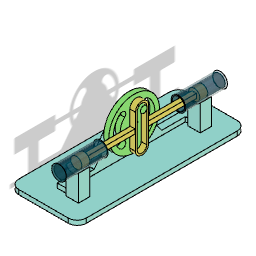
Scotch-Yoke_Mechanism (Autodesk Fusion 360 design; units mm, degrees)
Autodesk Fusion 360 part; units mm, degrees
note: some values were not read from the file. Set by a fixed rule: which sketch regions a step uses.
sketch "stand" plane through (0, 0, 0) normal (0, 0, 1) x (1, 0, 0) in component "holder stand"
  line L0 (75, 30) -> (-75, 30)
  line L1 (-75, 30) -> (-75, -30)
  line L2 (-75, -30) -> (75, -30)
  line L3 (75, -30) -> (75, 30)
  line L4 (75, 30) -> (-75, -30) construction
  line L5 (-75, 30) -> (75, -30) construction
  circle A0 centre (-61.0686, -17.8895) radius 7.5
  line L6 (0, 0) -> (75, 0)
  circle A1 centre (-61.0686, 17.8895) radius 7.5
  circle A2 centre (61.0686, 17.8895) radius 7.5
  circle A3 centre (61.0686, -17.8895) radius 7.5
  line L7 (20, 0) -> (-20, 0)
  line L8 (-20, 6) -> (20, 6)
  line L9 (-20, 0) -> (-30, 0)
  line L10 (-30, 0) -> (-30, 6)
  line L11 (-30, 6) -> (-20, 6)
  line L12 (20, 0) -> (30, 0)
  line L13 (30, 0) -> (30, 6)
  line L14 (30, 6) -> (20, 6)
  dimension "d1" = 150
  dimension "d2" = 60
  dimension "d3" = 15
  dimension "d10" = 40
  dimension "d11" = 6
  dimension "d16" = 40
  constraint horizontal L0
  constraint perpendicular L0 L1
  constraint parallel L0 L2
  constraint parallel L1 L3
  constraint coincident L4 L6.start
  constraint coincident L5 L6.start
  constraint midpoint L3 L6.end
  constraint symmetric A0 L6 A1
  constraint horizontal L7
  constraint horizontal L8
  constraint coincident L6 L7.start
  constraint horizontal L9
  constraint vertical L10
  constraint horizontal L11
  constraint horizontal L12
  constraint vertical L13
  constraint horizontal L14
  measures "d1" distance of L1.end L2.end
  measures "d2" distance of L0.end L1.end
  measures "d3" diameter of A0
  measures "d10" distance of L7.start L7.end
  measures "d11" distance of L7.start L8.end
  measures "d16" distance of L7.start L7.end
extrude "Extrude1" add sketch "stand" along normal blind 4 contours A0 | A1 | A2 | A3 makes body 1 at (68.5593, -18.2634, 2.6667) makes body 2 at (-53.5779, -18.2634, 2.6667) makes body 3 at (68.5593, 17.5157, 2.6667) makes body 4 at (-53.5779, 17.5157, 2.6667) in component "holder stand"
extrude "Extrude2" add sketch "stand" along normal blind 8 and the other way blind -4 contours L0 L1 L2 L3 | A0 | L6 L7 L8 L9 L10 L11 L12 L13 L14 | A1 | A2 | A3 bodies 1 2 3 4 in component "holder stand"
extrude "Extrude3" cut sketch "stand" along normal blind 50 contours L6 L7 L8 L9 L10 L11 L12 L13 L14 bodies 1 in component "holder stand"
fillet "Fillet1" radius 8 4 edges at (75, -30, 6) (-75, -30, 6) (75, 30, 6) (-75, 30, 6) on bodies 1 in component "holder stand"
sketch "holder" plane through (0, -6.0574, 0) normal (0, 1, 0) x (-1, 0, 0) in component "holder"
  line L0 (-30, 4) -> (30, 4)
  line L1 (30, 4) -> (30, 8)
  line L2 (30, 8) -> (-30, 8)
  line L3 (-30, 8) -> (-30, 4)
  line L4 (-30, 4) -> (30, 4)
  line L5 (30, 4) -> (30, 12)
  line L6 (30, 12) -> (-30, 12)
  line L7 (-30, 12) -> (-30, 4)
  line L8 (-30, 12) -> (-4.0576, 46.088)
  line L9 (30, 12) -> (4.0576, 46.088)
  arc A0 (4.0576, 46.088) -> (-4.0576, 46.088) centre (0, 43) ccw
  circle A1 centre (0, 35) radius 3
  line L10 (30, 12) -> (30, 8)
  line L11 (-30, 12) -> (-30, 4)
  dimension "d19" = 6
  constraint horizontal L4
  constraint vertical L5
  constraint horizontal L6
  constraint vertical L7
  constraint coincident L0.start L3.end
  constraint tangent L8 A0
  constraint coincident L1.end L2.start
  measures "d19" diameter of A1
extrude "Extrude1'" add sketch "holder" along normal blind 6 separate body contours L0 L1 L2 L3 L4 L5 L7 L11 | L2 L5 L6 L7 L10 L11 | L6 L8 L9 A0 | A1 makes body 5 in component "holder"
extrude "Extrude2'" add sketch "holder" along normal blind 12 contours A1 bodies 5 in component "holder"
sketch "crank" plane through (0, 5.9426, 0) normal (0, 1, 0) x (-1, 0, 0) in component "crank"
  circle A0 centre (0, 35) radius 3
  circle A1 centre (0, 35) radius 22.5
  circle A2 centre (0, 50) radius 3
  arc A3 (-8.4317, 44.0502) -> (-12.5322, 48.4516) centre (-10.4819, 46.2509) ccw
  arc A4 (-12.5322, 21.5484) -> (-8.4317, 25.9498) centre (-10.4819, 23.7491) ccw
  arc A5 (-8.4317, 44.0502) -> (-8.4317, 25.9498) centre (0, 35) ccw
  arc A6 (12.5322, 21.5484) -> (12.5322, 48.4516) centre (0, 35) ccw
  arc A7 (-12.5322, 48.4516) -> (-12.5322, 21.5484) centre (0, 35) ccw
  arc A8 (8.4317, 25.9498) -> (8.4317, 44.0502) centre (0, 35) ccw
  arc A9 (12.5322, 48.4516) -> (8.4317, 44.0502) centre (10.4819, 46.2509) ccw
  arc A10 (8.4317, 25.9498) -> (12.5322, 21.5484) centre (10.4819, 23.7491) ccw
  dimension "d22" = 45
  dimension "d23" = 6
  constraint concentric A0 A1
  constraint concentric A0 A5
  constraint concentric A1 A6
  constraint tangent A5 A9
  constraint coincident A3.end A6
  constraint concentric A5 A8
  constraint concentric A6 A7
  measures "d22" diameter of A1
  measures "d23" diameter of A2
extrude "Extrude1''" add sketch "crank" along normal blind -5 and the other way blind 0.5 separate body makes body 6 in component "crank"
extrude "Extrude2''" add sketch "crank" along normal blind 7 and the other way blind 5 contours A2 bodies 6 in component "crank"
sketch "slider" plane through (0, 5.4426, 0) normal (0, 1, 0) x (-1, 0, 0) in component "slider"
  arc A0 (-8.4317, 44.0502) -> (-12.5322, 48.4516) centre (-10.4819, 46.2509) ccw
  arc A1 (-8.4317, 44.0502) -> (-8.4317, 25.9498) centre (0, 35) ccw
  arc A2 (-12.5322, 21.5484) -> (-8.4317, 25.9498) centre (-10.4819, 23.7491) ccw
  arc A3 (-12.5322, 48.4516) -> (-12.5322, 21.5484) centre (0, 35) ccw
  arc A4 (8.4317, 25.9498) -> (12.5322, 21.5484) centre (10.4819, 23.7491) ccw
  arc A5 (8.4317, 25.9498) -> (8.4317, 44.0502) centre (0, 35) ccw
  arc A6 (12.5322, 48.4516) -> (8.4317, 44.0502) centre (10.4819, 46.2509) ccw
  arc A7 (12.5322, 21.5484) -> (12.5322, 48.4516) centre (0, 35) ccw
  circle A8 centre (0, 50) radius 3
  circle A9 centre (0, 35) radius 3
  circle A10 centre (0, 35) radius 22.5
  line L0 (-5.8308, 50.0372) -> (-5.831, 20)
  line L1 (5.831, 20) -> (5.831, 50)
  line L2 (4.2426, 20) -> (4.2426, 50)
  line L3 (-4.2426, 20) -> (-4.2426, 50)
  arc A11 (5.831, 50) -> (-5.8308, 49.9628) centre (0, 50) ccw
  arc A12 (4.2426, 50) -> (-4.2426, 50) centre (0, 50) ccw
  arc A13 (-5.831, 20) -> (5.831, 20) centre (0, 20) ccw
  arc A14 (-4.2426, 20) -> (4.2426, 20) centre (0, 20) ccw
  constraint concentric A8 A12
  constraint concentric A11 A12
  constraint coincident L0.start A11
  constraint tangent L0 A13
  constraint tangent L1 A11
  constraint vertical L1
  constraint tangent L2 A12
  constraint parallel L1 L2
  constraint tangent L3 A12
  constraint parallel L2 L3
  constraint coincident L0 A11.end
extrude "Extrude1'''" add sketch "slider" along normal blind 7 and the other way blind -2 separate body contours L0 L1 A11 A13 makes body 7 in component "slider"
sketch "slider right" plane through (-5.831, 0, 0) normal (-1, 0, 0) x (0, -1, 0) in component "slider"
  line L0 (-7.4426, 20) -> (-7.4426, 50)
  line L1 (-7.4426, 50) -> (-12.4426, 50)
  line L2 (-12.4426, 50) -> (-12.4426, 20)
  line L3 (-12.4426, 20) -> (-7.4426, 20)
  line L4 (-7.9426, 33) -> (-11.9426, 33)
  line L5 (-11.9426, 33) -> (-11.9426, 37)
  line L6 (-11.9426, 37) -> (-7.9426, 37)
  line L7 (-7.9426, 37) -> (-7.9426, 33)
  line L8 (-7.9426, 33) -> (-11.9426, 37) construction
  line L9 (-11.9426, 33) -> (-7.9426, 37) construction
  circle A0 centre (-9.9426, 35) radius 3
  dimension "d36" = 4
  dimension "d76" = 6
  constraint horizontal L4
  constraint perpendicular L4 L5
  constraint parallel L4 L6
  constraint parallel L5 L7
  constraint midpoint L9 A0.centre
  measures "d36" distance of L5.end L6.end
  measures "d76" diameter of A0
sketch "slider left" plane through (5.831, 0, 0) normal (1, 0, 0.000004) x (0, 1, 0) in component "slider"
  line L0 (7.4426, 50.0372) -> (7.4426, 20)
  line L1 (7.4426, 20) -> (12.4426, 20)
  line L2 (12.4426, 20) -> (12.4426, 50.0372)
  line L3 (12.4426, 50.0372) -> (7.4426, 50.0372)
  line L4 (11.9426, 33.0186) -> (7.9426, 33.0186)
  line L5 (7.9426, 33.0186) -> (7.9426, 37.0186)
  line L6 (7.9426, 37.0186) -> (11.9426, 37.0186)
  line L7 (11.9426, 37.0186) -> (11.9426, 33.0186)
  line L8 (11.9426, 33.0186) -> (7.9426, 37.0186) construction
  line L9 (7.9426, 33.0186) -> (11.9426, 37.0186) construction
  dimension "d37" = 4
  dimension "d38" = 4
  constraint horizontal L4
  constraint perpendicular L4 L5
  constraint parallel L4 L6
  constraint parallel L5 L7
  measures "d37" distance of L5.end L6.end
  measures "d38" distance of L4.end L5.end
extrude "Extrude2'''" add sketch "slider right" along normal blind 50 contours L4 L5 L6 L7 bodies 7 in component "slider"
extrude "Extrude3'" add sketch "slider left" along normal blind 50 contours L4 L5 L6 L7 bodies 7 in component "slider"
extrude "Extrude3''" add 1 faces at (0.5, 12.9426, 48.2662) along direction (0, 1, 0) blind 1 on bodies 6 bodies 6 in component "crank"
move_face "OffsetFaces1" offset -0.3 1 faces at (-2.9851, 1.9426, 35.2987) on bodies 5 in component "holder"
sketch "piston" plane through (5.831, 0, 0) normal (1, 0, 0.000004) x (0, 1, 0) in component "slider"
  line L0 (11.9426, 37.0186) -> (11.9426, 33.0186)
  line L1 (11.9426, 33.0186) -> (7.9426, 33.0186)
  line L2 (7.9426, 33.0186) -> (7.9426, 37.0186)
  line L3 (7.9426, 37.0186) -> (11.9426, 37.0186)
  line L4 (7.4426, 50.0372) -> (7.4426, 20)
  line L5 (7.4426, 20) -> (12.4426, 20)
  line L6 (12.4426, 20) -> (12.4426, 50.0372)
  line L7 (12.4426, 50.0372) -> (7.4426, 50.0372)
  circle A0 centre (9.9426, 35.0186) radius 3
  dimension "d71" = 6
  measures "d71" diameter of A0
extrude "Extrude4" add sketch "piston" along normal blind 50 and the other way blind -43 contours L0 L1 L2 L3 | L4 L6 A0 | L4 A0 | L6 A0 bodies 7 in component "slider"
extrude "Extrude5" add sketch "slider right" along normal blind 50 and the other way blind -43 contours L0 L2 A0 | L0 A0 | L2 A0 | L4 L5 L6 L7 bodies 7 in component "slider"
move_face "OffsetFaces1'" offset 2 1 faces at (53.4976, 12.9277, 35.3175) on bodies 7 in component "slider"
move_face "OffsetFaces2" offset 2 1 faces at (-51.1643, 6.9464, 35.1495) on bodies 7 in component "slider"
sketch "Sketch1" plane through (-55.7663, 0, 0) normal (-1, 0, 0) x (0, -1, 0) in component "right cylinder"
  circle A0 centre (-9.9426, 35) radius 5
  circle A1 centre (-9.9426, 35) radius 5.5
  circle A2 centre (-9.9426, 35) radius 6.5
  dimension "d84" = 11
  dimension "d85" = 13
  constraint concentric A0 A1
  constraint concentric A1 A2
  measures "d84" diameter of A1
  measures "d85" diameter of A2
extrude "Extrude1''''" add sketch "Sketch1" along normal blind 16 and the other way blind -15 separate body contours A0 makes body 8 in component "right cylinder"
extrude "Extrude2''''" add sketch "Sketch1" along normal blind 16 and the other way blind 21 separate body contours A2 makes body 9 in component "right cylinder"
extrude "Extrude3'''" add sketch "Sketch1" along normal blind 16 and the other way blind -15 contours A1 bodies 8 9 in component "right cylinder"
sketch "Sketch1 (2)" plane through (69.5884, 0, 0.0003) normal (1, 0, 0.000004) x (0, 1, 0) in component "left cylinder"
  circle A0 centre (9.9426, 35.0185) radius 5
extrude "Extrude1'''''" add 1 faces at (-34.7663, 3.8002, 34.6771) along direction (1, 0, 0) blind 106 and the other way blind -69 separate body on bodies 8 makes body 10 in component "left cylinder"
sketch "Sketch2" plane through (71.2337, 0, 0) normal (1, 0, 0) x (0, 1, 0) in component "left cylinder"
  circle A0 centre (9.9426, 35) radius 5.5
  circle A1 centre (9.9426, 35) radius 6.5
  circle A2 centre (9.9426, 35) radius 6.5
  constraint concentric A0 A2
extrude "Extrude2'''''" add sketch "Sketch2" against normal blind 1 contours A0 | A1 A2 bodies 10 in component "left cylinder"
sketch "Sketch5" plane through (0, 0, 8) normal (0, 0, 1) x (-1, 0, 0) in component "holder"
  arc A0 (-67, 30.0574) -> (-75, 22.0574) centre (-67, 22.0574) ccw
  line L0 (-75, 22.0574) -> (-75, -21.9426)
  arc A1 (-75, -21.9426) -> (-67, -29.9426) centre (-67, -21.9426) ccw
  line L1 (-67, -29.9426) -> (67, -29.9426)
  arc A2 (67, -29.9426) -> (75, -21.9426) centre (67, -21.9426) ccw
  line L2 (75, -21.9426) -> (75, 22.0574)
  arc A3 (75, 22.0574) -> (67, 30.0574) centre (67, 22.0574) ccw
  line L3 (67, 30.0574) -> (-67, 30.0574)
  line L4 (-30, 0.0574) -> (-30, 6.0574)
  line L5 (-30, 6.0574) -> (30, 6.0574)
  line L6 (30, 6.0574) -> (30, 0.0574)
  line L7 (30, 0.0574) -> (-30, 0.0574)
  line L8 (30, 0.0574) -> (50.8975, 0.0574)
  line L9 (56.8975, 0.0574) -> (56.8975, 6.0574)
  line L10 (56.8975, 6.0574) -> (30, 6.0574)
  line L11 (30, 6.0574) -> (30, 0.0574)
  line L12 (50.8975, 0.0574) -> (50.8975, -12.9426)
  line L13 (50.8975, -12.9426) -> (56.8975, -12.9426)
  line L14 (56.8975, -12.9426) -> (56.8975, 0.0574)
  line L15 (0, 6.0574) -> (0, 0)
  line L16 (-56.8975, 6.0574) -> (-30, 6.0574)
  line L17 (-30, 0.0574) -> (-50.8975, 0.0574)
  line L18 (-56.8975, 0.0574) -> (-56.8975, 6.0574)
  line L19 (-50.8975, 0.0574) -> (-50.8975, -12.9426)
  line L20 (-56.8975, -12.9426) -> (-56.8975, 0.0574)
  line L21 (-50.8975, -12.9426) -> (-56.8975, -12.9426)
  line L22 (-59, -15) -> (-49, -15)
  line L23 (-49, -15) -> (-49, -4)
  line L24 (-49, -4) -> (-59, -4)
  line L25 (-59, -4) -> (-59, -15)
  line L26 (0, -25) -> (0, -5)
  line L27 (49, -4) -> (59, -4)
  line L28 (49, -15) -> (49, -4)
  line L29 (59, -15) -> (49, -15)
  line L30 (59, -4) -> (59, -15)
  dimension "d107" = 6
  dimension "d108" = 13
  constraint horizontal L8
  constraint vertical L9
  constraint horizontal L10
  constraint vertical L11
  constraint coincident L6.end L7.start
  constraint vertical L12
  constraint horizontal L13
  constraint vertical L14
  constraint midpoint L5 L15.start
  constraint coincident L15.end origin
  constraint symmetric L6.end L15 L4.start
  constraint symmetric L9.start L15 L18.start
  constraint symmetric L9.end L15 L16.start
  constraint symmetric L5.end L15 L4.end
  constraint symmetric L8.end L15 L17.end
  constraint symmetric L12.end L15 L19.end
  constraint symmetric L13.end L15 L20.start
  constraint horizontal L22
  constraint vertical L23
  constraint horizontal L24
  constraint vertical L25
  constraint vertical L26
  constraint symmetric L22.start L26 L29.start
  constraint symmetric L22.end L26 L28.start
  constraint symmetric L23.end L26 L27.start
  constraint symmetric L24.end L26 L27.end
  measures "d107" distance of L9.start L8.end
  measures "d108" distance of L9.start L13.end
extrude "Extrude8" add sketch "Sketch5" along normal blind 4 contours L4 L16 L17 L18 L19 L20 L24 | L6 L8 L9 L10 L11 L12 L14 L27 | L19 L20 L21 L24 | L12 L13 L14 L27 bodies 5 in component "holder"
extrude "Extrude9" add sketch "Sketch5" along normal blind 25 contours L19 L20 L21 L22 L23 L24 L25 | L19 L20 L21 L24 bodies 5 in component "holder"
extrude "Extrude10" cut 1 faces at (71.2337, 12.9773, 34.3614) along direction (-1, 0, 0) blind 26 on bodies 10 bodies 5 in component "holder"
extrude "Extrude11" add sketch "Sketch5" along normal blind 25 contours L12 L13 L14 L27 | L12 L13 L14 L27 L28 L29 L30 bodies 5 in component "holder"
extrude "Extrude12" cut 1 faces at (-71.7663, 12.859, 35.9401) along direction (1, 0, 0) blind 25 on bodies 8 bodies 5 in component "holder"
component "holder stand" placed x (-1, 0, 0) y (0, -1, 0) z (0, 0, 1) at (0, -0.0574, 0)
component "holder" placed x (1, 0, 0) y (0, 1, 0) z (0, 0, 1) at (0, 0, 0)
component "crank" placed x (1, 0, 0) y (0, 1, 0) z (0, 0, 1) at (0, 0, 0)
component "slider" placed x (1, 0, 0) y (0, 1, 0) z (0, 0, 1) at (0.0647, 0, 0)
component "right cylinder" placed x (1, 0, 0) y (0, 1, 0) z (0, 0, 1) at (0, 0, 0)
component "left cylinder" placed x (1, 0, 0) y (0, 1, 0) z (0, 0, 1) at (0, 0, 0)
named bodies: "stand", "holder", "crank", "slider", "right cylinder", "left cylinder"
